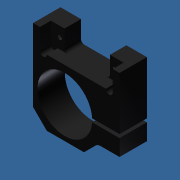
# Autodesk Inventor part: J002637
Saved by Autodesk Inventor 2012 SP2 (Build 160219200, 219)
## iProperties
Created: 2014-07-01
Material: ALUMINUM, 6061-T651
Vendor: HHMI: JFRC - ID&F
Document SubType Name: Modeling
Designer: NEGRASHOVI
Density: 2.7 g/cm^3
Part Number: J002637
Mass: 23.9941 g
Surface Area: 53.5778 cm^2
Volume: 8.88669 cm^3
Description: SPRING PIN PCB HOLDER
Project: P-159707
RuleStatus: InUse
AfterDocSave0: file://Part Number Cleaner
LAB/DEPT: RUBIN (LAB)
REQUESTING SCIENTIST: ASO, YOSHI
SURFACE ROUGHNESS: 32 Ra
DESIGN DEPARTMENT: HHMI: JFRC - ID&F
SPECIAL FINISH: ANODIZE PER MIL-A-8625F, TYPE II, CLASS 2 (BLACK)
ALTERED ITEM PART NUMBER: N/A
ALTERED ITEM VENDOR: N/A
ALTERED ITEM DESCRIPTION: N/A
Author: NEGRASHOVI
Revision Number: A
Autodesk Inventor part; units mm, degrees
note: some values were not read from the file. Chosen so that the rebuilt part matches the saved one: direction of "Hole2".
ref_plane "YZ Plane" through (0, 0, 0) normal (1, 0, 0) x (0, 1, 0)
ref_plane "XZ Plane" through (0, 0, 0) normal (0, 1, 0) x (-1, 0, 0)
ref_plane "XY Plane" through (0, 0, 0) normal (0, 0, 1) x (1, 0, 0)
sketch "Sketch1" plane through (0, 0, 0) normal (0, 0, 1) x (1, 0, 0)
  arc A0 (12.6748, 0.8001) -> (12.6748, -0.8001) centre (0, 0) ccw
  line L0 (-14.732, 25.4) -> (25.4, 25.4)
  line L1 (8.89, -14.732) -> (-8.382, -14.732)
  line L2 (-14.732, -8.382) -> (-14.732, 25.4)
  line L3 (-14.732, -8.382) -> (-8.382, -14.732)
  line L4 (8.89, -14.732) -> (15.24, -8.382)
  line L5 (15.24, -8.382) -> (25.4, -8.382)
  line L6 (-22.7584, 0) -> (33.4264, 0) construction
  line L7 (0, -22.7584) -> (0, 33.4264) construction
  line L8 (12.6748, 0.8001) -> (25.4, 0.8001)
  line L9 (12.6748, -0.8001) -> (25.4, -0.8001)
  line L10 (25.4, 25.4) -> (25.4, 0.8001)
  line L11 (25.4, -0.8001) -> (25.4, -8.382)
  dimension "d0" = 25.4
  dimension "d1" = 14.732
  dimension "d2" = 14.732
  dimension "d4" = 25.4
  dimension "d9" = 1.6002
  dimension "d11" = 45
  dimension "d12" = 25.4
  dimension "d14" = 8.89
  dimension "d15" = 15.24
  dimension "d49" = 45
  constraints: 20 end point, 6 perpendicular, 4 parallel, 2 point on circle, 1 centre point, 1 coincident, 1 collinear, 1 horizontal, 1 point on line, 1 other
  measures "d0" diameter of A0
  measures "d1" distance from line of L1 A0.centre
  measures "d2" distance from line of L2 point (0, 0)
  measures "d4" distance from line of L0 point (0, 0)
  measures "d9" distance between parallel lines of L9 L8
  measures "d11" angle of L4 L1
  measures "d12" distance between parallel lines of L11 L7
  measures "d14" distance from line of L1.start L7
  measures "d15" distance from line of L4.end L7
  measures "d49" angle of L3 L1
extrude "Extrusion1" add sketch "Sketch1" along normal blind 12.7
sketch "Sketch2" plane through (0, 0, 12.7) normal (0, 0, 1) x (1, 0, 0)
  line L0 (-14.732, -8.382) -> (-14.732, 25.4) projected
  line L1 (-14.732, 25.4) -> (25.4, 25.4) projected
  line L2 (25.4, 25.4) -> (25.4, 0.8001) projected
  line L3 (-22.7584, 0) -> (33.4264, 0) construction
  line L4 (0, -22.7584) -> (0, 33.4264) construction
  line L5 (-11.557, 25.4) -> (22.225, 25.4)
  line L6 (22.225, 25.4) -> (22.225, 15.875)
  line L7 (19.05, 15.875) -> (-8.382, 15.875)
  line L8 (-11.557, 15.875) -> (-11.557, 25.4)
  arc A0 (-11.557, 15.875) -> (-8.382, 15.875) centre (-9.9695, 15.875) ccw
  arc A1 (19.05, 15.875) -> (22.225, 15.875) centre (20.6375, 15.875) ccw
  point P0 (0, 0)
  dimension "d16" = 3.175
  dimension "d17" = 3.175
  dimension "d18" = 9.525
  dimension "d19" = 3.175
  constraints: 8 end point, 4 point on circle, 3 point on line, 2 centre point, 2 parallel, 2 tangent, 1 equal radius, 1 horizontal, 1 perpendicular
  measures "d16" distance between parallel lines of L8 L0
  measures "d17" distance between parallel lines of L2 L6
  measures "d18" distance between parallel lines of L7 L1
  measures "d19" diameter of A0
extrude "Extrusion2" cut sketch "Sketch2" against normal blind 5.08
sketch "Sketch3" plane through (0, 0, 7.62) normal (0, 0, 1) x (1, 0, 0)
  line L0 (-11.557, 25.4) -> (22.225, 25.4) projected
  line L1 (-8.382, 15.875) -> (19.05, 15.875) projected
  line L2 (-5.207, 25.4) -> (15.875, 25.4)
  line L3 (15.875, 25.4) -> (15.875, 17.4752)
  line L4 (14.2748, 15.875) -> (-3.6068, 15.875)
  line L5 (-5.207, 17.4752) -> (-5.207, 25.4)
  arc A0 (-5.207, 17.4752) -> (-3.6068, 15.875) centre (-3.6068, 17.4752) ccw
  arc A1 (14.2748, 15.875) -> (15.875, 17.4752) centre (14.2748, 17.4752) ccw
  line L6 (5.334, 25.4) -> (5.334, 15.875) construction
  point P0 (0, 0)
  point P1 (15.875, 15.875)
  dimension "d22" = 1.6002
  dimension "d24" = 6.35
  constraints: 10 end point, 4 point on circle, 4 point on line, 4 tangent, 2 centre point, 2 midpoint, 2 parallel, 1 equal radius, 1 horizontal, 1 perpendicular, 1 other
  measures "d22" radius of A0
  measures "d24" distance from line of L5 L0.start
extrude "Extrusion3" cut sketch "Sketch3" against normal through all
sketch "Sketch4" plane through (0, 0, 7.62) normal (0, 0, 1) x (1, 0, 0)
  line L0 (22.225, 25.4) -> (22.225, 15.875) projected
  line L1 (-11.557, 25.4) -> (-11.557, 15.875) projected
  line L2 (-11.557, 20.6375) -> (22.225, 20.6375) construction
  line L3 (5.334, 29.021) -> (5.334, 12.254) construction
  point P0 (0, 0)
  point P1 (-7.366, 20.6375)
  point P2 (18.034, 20.6375)
  point P3 (23.8317, 40.0005)
  point P4 (5.334, 20.6375)
  dimension "d27" = 25.4
  constraints: 4 end point, 4 midpoint, 2 point on line, 1 perpendicular, 1 symmetric about line
  measures "d27" distance of point (18.034, 20.637) point (-7.366, 20.637)
hole "Hole1" at (-7.366, 20.6375, 7.62) at (18.034, 20.6375, 7.62) at (23.8317, 40.0005, 7.62) direction (0, 0, -1) diameter 1.7018 end through all
sketch "Sketch5" plane through (15.24, -8.382, 0) normal (0, -1, 0) x (1, 0, 0)
  line L0 (10.16, 12.7) -> (0, 12.7) projected
  line L1 (0, 0) -> (0, 12.7) projected
  line L2 (10.16, 0) -> (0, 0) projected
  line L3 (10.16, 0) -> (10.16, 12.7) projected
  line L4 (5.08, 12.7) -> (5.08, 0) construction
  point P0 (-15.24, 0)
  point P1 (5.08, 6.35)
  constraints: 3 midpoint, 2 end point
hole "Hole2" at (20.32, -8.382, 6.35) direction (0, 1, 0) diameter 4.4958 end up to surface counterbore diameter 7.9502 counterbore depth 4.1656 clearance for "Socket Head Cap Screw" size "#8" standard "Ansi Unified Screw Threads"
sketch "Sketch6" plane through (12.6748, 0.8001, 0) normal (0, -1, 0) x (1, 0, 0)
  circle A0 centre (7.6452, 6.35) radius 2.2479 projected
  point P0 (-12.6748, 0)
  constraints: 1 coincident
hole "Hole3" at (20.32, 0.8001, 6.35) direction (0, 1, 0) diameter 3.302 depth 10.16 tip angle 118 thread size "8-32 UNC" class "2B" standard "ANSI Unified Screw Threads"
fillet "Fillet1" radius 3.175 1 edges at (15.24, -8.382, 6.35)
equation "\"d1\" = d2"
equation "\"d14\" = d13"
equation "\"d17\" = d16"
equation "\"d13\" = 8.89"
body "Solid1"
